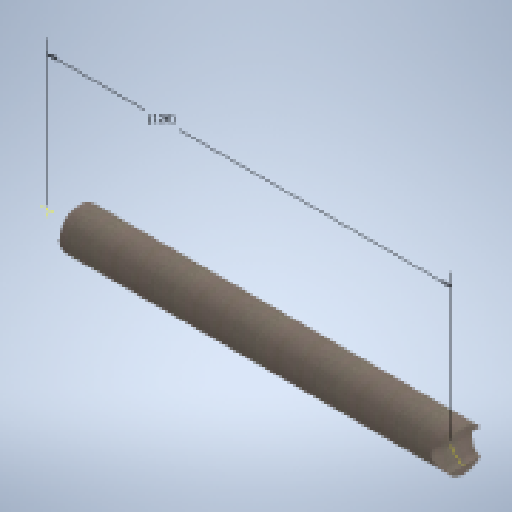
# Autodesk Inventor part: Short Arm
Saved by Autodesk Inventor 2025.2 (Build 292293000, 293)
## iProperties
Created: 2025-02-17
Part Number: Short Arm
Material: Wood (Oak)
Document SubType Name: Modeling
Designer: baolo
Density: 0.76 g/cm^3
Appearance: Walnut
Mass: 56.5536 g
Surface Area: 160.867 cm^2
Volume: 74.4126 cm^3
Author: baolo
Autodesk Inventor part; units mm, degrees
ref_plane "YZ Plane" through (0, 0, 0) normal (1, 0, 0) x (0, 1, 0)
ref_plane "XZ Plane" through (0, 0, 0) normal (0, 1, 0) x (-1, 0, 0)
sketch "Sketch1" plane through (0, 0, 0) normal (1, 0, 0) x (0, 1, 0)
  circle A0 centre (0, 0) radius 6.35
  circle A1 centre (0, 0) radius 6.35 construction
  constraints: 1 centre point, 1 coincident, 1 concentric
extrude "Extrusion1" add sketch "Sketch1" along normal blind 120
ref_plane "Work Plane1" through (0, 0, 6.35) normal (0, 0, 1) x (1, 0, 0)
sketch "Sketch2" plane through (0, 0, 6.35) normal (0, 0, 1) x (1, 0, 0)
  line L0 (120, -6.35) -> (120, 6.35) construction
  line L1 (-38, 0) -> (158, 0) construction
  line L2 (0, -6.35) -> (0, 6.35) projected
  point P0 (0, 0)
  point P1 (120, 0)
  dimension "d11" = 120
  constraints: 1 point on line
  measures "d11" distance from line of L2 point (120, 0)
hole "Hole1" at (120, 0, 6.35) direction (0, 0, -1) diameter 8 end through all
sketch "Sketch3" plane through (0, 0, 0) normal (0, 0, 1) x (1, 0, 0)
  point P0 (0, 0)
  point P1 (-10, 0)
  point P2 (116, 0)
  dimension "d13" = 126
  constraints: 1 other
  measures "d13" distance of point (-10, 0) point (116, 0)
equation "\"d1\" = ShortArmLen"
equation "\"d11\" = ShortArmLen"
equation "\"ShortArmLen\" = 120"
body "Solid1"
